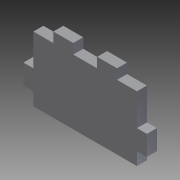
# Autodesk Inventor part: support 2
Saved by Autodesk Inventor 2011 (Build 150239000, 239)
## iProperties
Created: 2011-02-21
Part Number: support 2
Document SubType Name: Modeling
Designer: adowning
Density: 1 g/cm^3
Author: adowning
Autodesk Inventor part; units mm, degrees
ref_plane "YZ Plane" through (0, 0, 0) normal (1, 0, 0) x (0, 1, 0)
ref_plane "XZ Plane" through (0, 0, 0) normal (0, 1, 0) x (-1, 0, 0)
ref_plane "XY Plane" through (0, 0, 0) normal (0, 0, 1) x (1, 0, 0)
sketch "Sketch1" plane through (0, 0, 0) normal (0, 0, 1) x (1, 0, 0)
  line L0 (-18.7161, 14.4213) -> (-18.7161, -26.8537)
  line L1 (-18.7161, 14.4213) -> (47.3239, 14.4213)
  line L2 (47.3239, 14.4213) -> (47.3239, -26.8537)
  line L3 (47.3239, -26.8537) -> (-18.7161, -26.8537)
  line L4 (-18.7161, 14.4213) -> (-6.0161, 14.4213)
  line L5 (-6.0161, 14.4213) -> (-6.0161, 20.7713)
  line L6 (-6.0161, 20.7713) -> (6.6839, 20.7713)
  line L7 (6.6839, 20.7713) -> (6.6839, 14.4213)
  line L8 (47.3239, 14.4213) -> (34.6239, 14.4213)
  line L9 (34.6239, 14.4213) -> (34.6239, 20.7713)
  line L10 (34.6239, 20.7713) -> (21.9239, 20.7713)
  line L11 (21.9239, 20.7713) -> (21.9239, 14.4213)
  line L12 (-18.7161, 14.4213) -> (-18.7161, -5.8987)
  line L13 (-18.7161, -5.8987) -> (-25.0661, -5.8987)
  line L14 (-25.0661, -5.8987) -> (-25.0661, -18.5987)
  line L15 (-25.0661, -18.5987) -> (-18.7161, -18.5987)
  line L16 (47.3239, 14.4213) -> (47.3239, -5.8987)
  line L17 (47.3239, -5.8987) -> (53.6739, -5.8987)
  line L18 (53.6739, -5.8987) -> (53.6739, -18.5987)
  line L19 (53.6739, -18.5987) -> (47.3239, -18.5987)
  point P0 (0, 0)
  dimension "d0" = 41.275
  dimension "d1" = 66.04
  dimension "d2" = 12.7
  dimension "d3" = 6.35
  dimension "d4" = 12.7
  dimension "d5" = 12.7
  dimension "d6" = 12.7
  dimension "d7" = 20.32
  dimension "d8" = 6.35
  dimension "d9" = 12.7
  dimension "d10" = 20.32
  dimension "d11" = 6.35
  constraints: 40 end point, 12 perpendicular, 8 point on line, 3 parallel, 1 vertical
  measures "d0" distance of L0.start L0.end
  measures "d1" distance of L0.start L1.end
  measures "d2" distance of L0.start L4.end
  measures "d3" distance of L4.end L5.end
  measures "d4" distance of L5.end L6.end
  measures "d5" distance of L1.end L8.end
  measures "d6" distance of L9.end L10.end
  measures "d7" distance of L0.start L12.end
  measures "d8" distance of L12.end L13.end
  measures "d9" distance of L13.end L14.end
  measures "d10" distance of L1.end L16.end
  measures "d11" distance of L16.end L17.end
extrude "Extrusion1" add sketch "Sketch1" along normal blind 6.35
body "Solid1"
